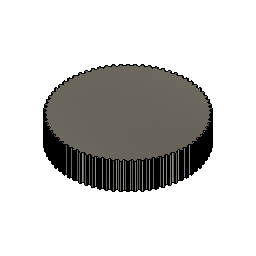
gear_72 (Autodesk Fusion 360 design; units mm, degrees)
Autodesk Fusion 360 part; units mm, degrees
sketch "Sketch1" plane through (0, 0, 0) normal (0, 0, 1) x (1, 0, 0) in component "gt2 pulley"
  circle A0 centre (0, 0) radius 22.9183 construction
  circle A1 centre (0, 0) radius 21.9143 construction
  line L0 (0, 0) -> (0, 22.9183) construction
  line L1 (0, 0) -> (0.9997, 22.8965) construction
  line L2 (0, 0) -> (1.4054, 22.8752) construction
  circle A2 centre (0, 0) radius 22.6643 construction
  arc A3 (0.3943, 22.5272) -> (0.4691, 22.2312) centre (1.3898, 22.6217) ccw
  circle A4 centre (0, 0) radius 22.5143 construction
  arc A5 (0.2465, 22.663) -> (0, 22.6643) centre (0, 0) ccw
  arc A6 (0.3943, 22.5272) -> (0.2465, 22.663) centre (0.2449, 22.513) ccw
  arc A7 (0.4691, 22.2312) -> (0.9559, 21.8935) centre (0.9801, 22.4479) ccw
  arc A8 (0, 22.6643) -> (-0.2465, 22.663) centre (0, 0) ccw
  arc A9 (-0.2465, 22.663) -> (-0.3943, 22.5272) centre (-0.2449, 22.513) ccw
  arc A10 (-0.4691, 22.2312) -> (-0.3943, 22.5272) centre (-1.3898, 22.6217) ccw
  arc A11 (-0.9559, 21.8935) -> (-0.4691, 22.2312) centre (-0.9801, 22.4479) ccw
  arc A12 (0.9559, 21.8935) -> (-0.9559, 21.8935) centre (0, 0) ccw
  point P0 (1.3898, 22.6217)
  point P1 (0, 22.6643)
  dimension "d18" = 45.8366
  dimension "d19" = 2.5
  dimension "d22" = 1.004
  dimension "d24" = 0.75
  dimension "d26" = 1
  dimension "d27" = 0.15
  dimension "d28" = 0.15
  dimension "d47" = 0.555
  dimension "d52" = 3.812
  constraint coincident A0.centre A1.centre
  constraint coincident A0 L0.end
  constraint vertical L0
  constraint coincident A0 L1.end
  constraint coincident A0 L2.end
  constraint concentric A1 A2
  constraint coincident A1 A7.end
  constraint coincident L1 A7.end
  constraint coincident A2 P0
  constraint coincident L2 P0
  constraint coincident P0 A3.centre
  constraint coincident A2 P1
  constraint coincident L0 P1
  constraint concentric A2 A4
  constraint coincident P1 A5.end
  constraint coincident A4 A6.centre
  constraint coincident A3.start A6.start
  constraint tangent A3 A6
  constraint tangent A3 A7
  constraint symmetric L0 A7.end A11.start
  constraint symmetric L0 A3.start A9.end
  constraint symmetric L0 A3.end A10.start
  constraint symmetric L0 A3 A10
  constraint symmetric L0 A5.start A8.end
  constraint symmetric L0 P1 A5.end
  constraint symmetric L0 A5 A8
  constraint symmetric L0 A6 A9
  constraint symmetric L0 A7 A11
  constraint coincident A1 A11.start
  constraint tangent A1 A7
  constraint coincident L1 A7.centre
  measures "d18" diameter of A0
  measures "d19" angle of L0 L1
  measures "d22" distance of A0 A1
  measures "d24" distance of A1 A2
  measures "d26" radius of A3
  measures "d27" distance of A2 A4
  measures "d28" radius of A6
  measures "d47" radius of A7
extrude "Extrude1" add sketch "Sketch1" along normal blind 10 makes body 1
pattern_circular "C-Pattern1" count 72 over 360 about axis through (0, 0, 1.75) along (0, 0, 1) of bodies 1 makes body 2 at (-2.6496, 21.7535, 6.6667) makes body 3 at (-3.0709, 21.6981, 6.6667) makes body 4 at (-5.7744, 21.1399, 6.6667) makes body 5 at (-6.7921, 20.8352, 3.3333) makes body 6 at (-8.5822, 20.1639, 6.6667) makes body 7 at (-11.5948, 18.5956, 6.6667) makes body 8 at (-12.6564, 17.89, 6.6667) makes body 9 at (-13.5085, 17.2556, 3.3333) makes body 10 at (-15.5707, 15.4205, 6.6667) makes body 11 at (-16.8554, 14.0047, 6.6667) makes body 12 at (-17.5143, 13.1714, 3.3333) makes body 13 at (-19.3392, 10.3069, 6.6667) makes body 14 at (-19.9058, 9.165, 6.6667) makes body 15 at (-20.6288, 7.3952, 6.6667) makes body 16 at (-21.1948, 5.5692, 6.6667) makes body 17 at (-21.4398, 4.5355, 3.3333) makes body 18 at (-21.7535, 2.6496, 3.3333) makes body 19 at (-21.9017, -0.7436, 6.6667) makes body 20 at (-21.8832, -1.1681, 3.3333) makes body 21 at (-21.6981, -3.0709, 6.6667) makes body 22 at (-21.1399, -5.7744, 6.6667) makes body 23 at (-20.8352, -6.7921, 3.3333) makes body 24 at (-20.1639, -8.5822, 6.6667) makes body 25 at (-18.5956, -11.5948, 6.6667) makes body 26 at (-18.3673, -11.9532, 3.3333) makes body 27 at (-17.2556, -13.5085, 3.3333) makes body 28 at (-15.4205, -15.5707, 6.6667) makes body 29 at (-13.5085, -17.2556, 6.6667) makes body 30 at (-13.1714, -17.5143, 3.3333) makes body 31 at (-11.5948, -18.5956, 3.3333) makes body 32 at (-9.165, -19.9058, 6.6667) makes body 33 at (-7.3952, -20.6288, 6.6667) makes body 34 at (-6.3868, -20.963, 3.3333) makes body 35 at (-4.5355, -21.4398, 6.6667) makes body 36 at (-2.6496, -21.7535, 3.3333) makes body 37 at (-0.7436, -21.9017, 3.3333) makes body 38 at (2.6496, -21.7535, 6.6667) makes body 39 at (3.7007, -21.5996, 6.6667) makes body 40 at (5.7744, -21.1399, 6.6667) makes body 41 at (7.5949, -20.5561, 6.6667) makes body 42 at (8.5822, -20.1639, 6.6667) makes body 43 at (10.3069, -19.3392, 3.3333) makes body 44 at (11.9532, -18.3673, 3.3333) makes body 45 at (13.5085, -17.2556, 3.3333) makes body 46 at (16.0126, -14.9611, 6.6667) makes body 47 at (17.2556, -13.5085, 6.6667) makes body 48 at (17.5143, -13.1714, 3.3333) makes body 49 at (19.3392, -10.3069, 6.6667) makes body 50 at (19.9058, -9.165, 6.6667) makes body 51 at (20.6288, -7.3952, 6.6667) makes body 52 at (21.1948, -5.5692, 6.6667) makes body 53 at (21.4398, -4.5355, 6.6667) makes body 54 at (21.7535, -2.6496, 3.3333) makes body 55 at (21.9017, -0.7436, 3.3333) makes body 56 at (21.7535, 2.6496, 6.6667) makes body 57 at (21.5996, 3.7007, 6.6667) makes body 58 at (21.1399, 5.7744, 6.6667) makes body 59 at (20.5561, 7.5949, 6.6667) makes body 60 at (20.1639, 8.5822, 6.6667) makes body 61 at (19.3392, 10.3069, 3.3333) makes body 62 at (17.89, 12.6564, 6.6667) makes body 63 at (17.2556, 13.5085, 3.3333) makes body 64 at (15.4205, 15.5707, 6.6667) makes body 65 at (13.5085, 17.2556, 6.6667) makes body 66 at (13.1714, 17.5143, 3.3333) makes body 67 at (10.3069, 19.3392, 6.6667) makes body 68 at (9.165, 19.9058, 6.6667) makes body 69 at (8.1895, 20.3265, 3.3333) makes body 70 at (5.5692, 21.1948, 6.6667) makes body 71 at (4.5355, 21.4398, 6.6667) makes body 72 at (2.6496, 21.7535, 3.3333)
sketch "Sketch2" plane through (0, 0, 10) normal (0, 0, 1) x (-1, 0, 0)
  arc A0 (-9.8777, -20.2499) -> (-9.8012, -20.4355) centre (-9.7364, -20.3002) ccw
  arc A1 (-9.8012, -20.4355) -> (-9.3544, -20.6438) centre (0, 0) ccw
  arc A2 (-9.3544, -20.6438) -> (-9.1631, -20.5832) centre (-9.2924, -20.5072) ccw
  arc A3 (-8.9701, -20.3466) -> (-9.1631, -20.5832) centre (-8.3008, -21.0895) ccw
  arc A4 (-8.3862, -20.2462) -> (-8.9701, -20.3466) centre (-8.5986, -20.7589) ccw
  arc A5 (-10.1189, -19.4382) -> (-8.3862, -20.2462) centre (0, 0) ccw
  arc A6 (-9.8205, -19.9501) -> (-10.1189, -19.4382) centre (-10.3752, -19.9305) ccw
  arc A7 (-9.8777, -20.2499) -> (-9.8205, -19.9501) centre (-10.8199, -19.9148) ccw
  circle A8 centre (0, 0) radius 21.9143
  constraint coincident A1.centre A5.centre
extrude "Extrude2" add sketch "Sketch2" against normal blind 10 contours A5 A8 bodies 1 2 3 4 5 6 7 8 9 10 11 12 13 14 15 16 17 18 19 20 21 22 23 24 25 26 27 28 29 30 31 32 33 34 35 36 37 38 39 40 41 42 43 44 45 46 47 48 49 50 51 52 53 54 55 56 57 58 59 60 61 62 63 64 65 66 67 68 69 70 71 72
extrude "Extrude4" [suppressed] in component "gt2 pulley"
pattern_circular "C-Pattern7" [suppressed] in component "gt2 pulley"
extrude "Extrude3" [suppressed] in component "gt2 pulley"
pattern_circular "C-Pattern6" [suppressed] in component "gt2 pulley"
extrude "Extrude2'" [suppressed] in component "gt2 pulley"
pattern_circular "C-Pattern5" [suppressed] in component "gt2 pulley"
extrude "Extrude1'" [suppressed] in component "gt2 pulley"
pattern_circular "C-Pattern4" [suppressed] in component "gt2 pulley"
pattern_circular "C-Pattern3" [suppressed] in component "gt2 pulley"
pattern_circular "C-Pattern2" [suppressed] in component "gt2 pulley"
pattern_circular "C-Pattern1'" [suppressed] in component "gt2 pulley"
copy_body "Body->Comp1" [suppressed] in component "Component"
copy_body "Body->Comp2" [suppressed] in component "Component'"
copy_body "Body->Comp3" [suppressed] in component "Component''"
copy_body "Body->Comp4" [suppressed] in component "Component'''"
copy_body "Body->Comp5" [suppressed] in component "Component''''"
copy_body "Body->Comp6" [suppressed] in component "Component'''''"
copy_body "Body->Comp7" [suppressed] in component "Component''''''"
copy_body "Body->Comp8" [suppressed] in component "Component'''''''"
copy_body "Body->Comp9" [suppressed] in component "Component''''''''"
copy_body "Body->Comp10" [suppressed] in component "Component'''''''''"
copy_body "Body->Comp11" [suppressed] in component "Component''''''''''"
copy_body "Body->Comp12" [suppressed] in component "Component'''''''''''"
copy_body "Body->Comp13" [suppressed] in component "Component''''''''''''"
copy_body "Body->Comp14" [suppressed] in component "Component'''''''''''''"
copy_body "Body->Comp15" [suppressed] in component "Component''''''''''''''"
copy_body "Body->Comp16" [suppressed] in component "Component'''''''''''''''"
copy_body "Body->Comp17" [suppressed] in component "Component''''''''''''''''"
copy_body "Body->Comp18" [suppressed] in component "Component'''''''''''''''''"
copy_body "Body->Comp19" [suppressed] in component "Component''''''''''''''''''"
copy_body "Body->Comp20" [suppressed] in component "Component'''''''''''''''''''"
component "gt2 pulley" placed x (1, 0, 0) y (0, 1, 0) z (0, 0, 1) at (0, 0, 0)
equation "NumTeeth = 72" comment "min 20"
equation "ToothPitch = 2 mm"
equation "PullyDia = NumTeeth * ToothPitch / PI"
equation "ToothAng = ( ( 360 / NumTeeth ) * 1 deg )"
equation "TransOffsetAngle = ToothAng * 0.2"
equation "Sholulder_Radius = 0.15 mm"
equation "Root_Radius = 0.555 mm"
equation "TransRadius = 1 mm"
equation "ToolHeight = 0.75 mm"
equation "PLD = 0.254 mm"
equation "d18 = PullyDia"
equation "d19 = ToothAng / 2"
equation "d22 = PLD + ToolHeight"
equation "d24 = ToolHeight"
equation "d26 = TransRadius"
equation "d27 = Sholulder_Radius"
equation "d31 = NumTeeth"
equation "d33 = NumTeeth"
equation "d35 = NumTeeth"
equation "d37 = NumTeeth"
equation "d41 = NumTeeth"
equation "d45 = NumTeeth"
equation "d47 = Root_Radius"
equation "d50 = NumTeeth"
